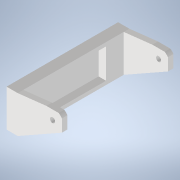
# Autodesk Inventor part: Part6
Saved by Autodesk Inventor 2022 (Build 260153000, 153)
## iProperties
Created: 2024-04-11
Part Number: Part6
Material: Generic
Document SubType Name: Modeling
Designer: Gotham City
Density: 1 g/cm^3
Appearance: Default
Author: Gotham City
Autodesk Inventor part; units mm, degrees
ref_plane "YZ Plane" through (0, 0, 0) normal (1, 0, 0) x (0, 1, 0)
ref_plane "XZ Plane" through (0, 0, 0) normal (0, 1, 0) x (-1, 0, 0)
ref_plane "Work Plane1" through (4.77, 2.8444, 22.011) normal (0, 0, 1) x (1, 0, 0)
sketch "Sketch1" plane through (0, 0, 0) normal (0, 0, 1) x (1, 0, 0)
  line L0 (0.5, -10) -> (-5.5, -10)
  line L1 (-5.5, -10) -> (-5.5, 10)
  line L2 (-5.5, 10) -> (0.5, 10)
  line L3 (0.5, 10) -> (0.5, -10)
  line L4 (-4, 8) -> (-4, -8) construction
  line L5 (0, 8) -> (-4, 8) construction
  line L6 (0, -8) -> (-4, -8) construction
  line L7 (0.5, -14.6916) -> (0.5, 15.0789) construction
  point P0 (0, 0)
  dimension "d0" = 2
  dimension "d1" = 2
  dimension "d3" = 6
  dimension "d4" = 0
  constraints: 10 end point, 2 parallel, 1 horizontal, 1 perpendicular, 1 vertical, 2 other
  measures "d0" distance between parallel lines of L0 L6
  measures "d1" distance between parallel lines of L2 L5
  measures "d3" distance of L1.end L2.end
  measures "d4" distance between parallel lines of L7 L3
extrude "Extrusion1" add sketch "Sketch1" along normal mid plane 60
sketch "Sketch2" plane through (0.5, -10, 30) normal (1, 0, 0) x (0, 0, -1)
  line L0 (47.5, 18) -> (12.5, 18) projected
  line L1 (12.5, 18) -> (12.5, 2) projected
  line L2 (12.5, 2) -> (47.5, 2) projected
  line L3 (47.5, 2) -> (47.5, 18) projected
  line L4 (41.725, 8.15) -> (18.275, 8.15) projected
  arc A0 (17.675, 8.75) -> (18.275, 8.15) centre (18.275, 8.75) ccw projected
  line L5 (17.675, 8.75) -> (17.675, 11.25) projected
  arc A1 (18.275, 11.85) -> (17.675, 11.25) centre (18.275, 11.25) ccw projected
  line L6 (18.275, 11.85) -> (41.725, 11.85) projected
  arc A2 (42.325, 11.25) -> (41.725, 11.85) centre (41.725, 11.25) ccw projected
  line L7 (42.325, 11.25) -> (42.325, 8.75) projected
  arc A3 (41.725, 8.15) -> (42.325, 8.75) centre (41.725, 8.75) ccw projected
  point P0 (30, 10)
extrude "Extrusion2" cut sketch "Sketch2" against normal blind 4 contours L3 L2 L1 L0 | L4 A0 L5 A1 L6 A2 L7 A3
sketch "Sketch3" plane through (0, 0, 30) normal (0, 0, 1) x (1, 0, 0)
  arc A0 (13.2615, 6.3791) -> (13.2616, 6.3779) centre (19.25, 6.75) ccw construction
  line L0 (-5.5, -10) -> (0.5, -10) projected
  line L1 (0.5, 10) -> (-5.5, 10) projected
  line L2 (0.5, 10) -> (0.5, -10)
  circle A1 centre (19.25, 6.75) radius 1.375
  line L3 (4.77, 6.75) -> (24.4771, 6.75) construction
  line L4 (24.25, 3.4334) -> (24.25, 10.0666)
  line L5 (22.5666, 11.75) -> (15.9334, 11.75)
  line L6 (24.25, 6.75) -> (19.25, 6.75) construction
  line L7 (19.25, 11.75) -> (19.25, 6.75) construction
  arc A2 (18.6093, 0.7843) -> (22.5666, 11.75) centre (19.25, 6.75) ccw
  line L8 (15.9334, 11.75) -> (0.5, 10)
  line L9 (0.5, -10) -> (24.25, 3.4334)
  arc A3 (2.5, 31.5) -> (-5.5, -10) centre (19.25, 6.75) ccw construction
  line L10 (0.5, -10) -> (0.5, 10) construction
  arc A4 (2.5, 25.5) -> (0.5, -10) centre (19.25, 6.75) ccw construction
  line L11 (2.5, 31.5) -> (2.5, 25.5) construction
  line L12 (2.77, 3.75) -> (0.5, 3.75) construction
  point P0 (0, 0)
  point P1 (19.25, 12.75)
  dimension "d12" = 2.75
  dimension "d13" = 6
  dimension "d18" = 1
  dimension "d19" = 2
  dimension "d20" = 3
  constraints: 18 end point, 14 point on circle, 5 centre point, 5 perpendicular, 4 coincident, 3 point on line, 2 midpoint, 2 vertical, 1 concentric, 1 horizontal, 1 vertical alignment
  measures "d12" diameter of A1
  measures "d13" radius of A0
  measures "d18" distance of L7.start point (19.25, 12.75)
  measures "d19" distance between parallel lines of L2 L11
  measures "d20" distance between parallel lines of L12 L3
extrude "Extrusion3" add sketch "Sketch3" against normal blind 3 contours L8 L5 A2 L4 L9 L2
mirror "Mirror1" about plane through (0, 0, 0) normal (0, 0, 1) of "Extrusion3"
body "Solid1"
